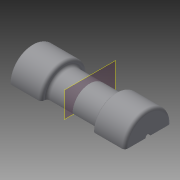
# Autodesk Inventor part: resistor
Saved by Autodesk Inventor 2015 (Build 190159000, 159)
## iProperties
Created: 2014-08-01
Part Number: resistor
Material: Generic
Document SubType Name: Modeling
Designer: dan
Density: 1 g/cm^3
Appearance: Default
Author: dan
Autodesk Inventor part; units mm, degrees
ref_plane "XZ Plane" through (0, 0, 0) normal (0, 1, 0) x (-1, 0, 0)
ref_plane "XY Plane" through (0, 0, 0) normal (0, 0, 1) x (1, 0, 0)
sketch "Sketch1" plane through (0, 0, 0) normal (0, 1, 0) x (-1, 0, 0)
  line L0 (0, 0) -> (0, -12.7)
  line L1 (0, -12.7) -> (-17.78, -12.7)
  line L2 (-17.78, -12.7) -> (-17.78, -9.525)
  line L3 (-17.78, -9.525) -> (-45.72, -9.525)
  line L4 (-45.72, -9.525) -> (-45.72, -12.7)
  line L5 (-45.72, -12.7) -> (-63.5, -12.7)
  line L6 (-63.5, -12.7) -> (-63.5, 0)
  line L7 (-63.5, 0) -> (-60.325, 0)
  line L8 (-60.325, 0) -> (-60.325, -6.35)
  line L9 (-60.325, -6.35) -> (-3.175, -6.35)
  line L10 (-3.175, -6.35) -> (-3.175, 0)
  line L11 (-3.175, 0) -> (0, 0)
  dimension "d0" = 12.7
  dimension "d1" = 3.175
  dimension "d2" = 17.78
  dimension "d3" = 63.5
  dimension "d4" = 3.175
  dimension "d5" = 3.175
  constraints: 24 end point, 10 perpendicular, 3 point on line, 2 collinear, 1 vertical
  measures "d0" distance of L0.start L0.end
  measures "d1" distance of L1.end L2.end
  measures "d2" distance of L0.end L1.end
  measures "d3" distance between parallel lines of L6 L0
  measures "d4" distance between parallel lines of L3 L9
  measures "d5" distance of L10.end L0.start
revolve "Revolution1" add sketch "Sketch1" angle 180 about axis through (63.5, 0, 0) along (1, 0, 0)
fillet "Fillet1" radius 1.5875 6 edges at (63.5, 12.7, 0) (17.78, 9.525, 0) (17.78, 12.7, 0) (0, 12.7, 0) (45.72, 9.525, 0) (45.72, 12.7, 0)
sketch "Sketch2" plane through (0, 0, 0) normal (-1, 0, 0) x (0, 0, 1)
  circle A0 centre (0, 0) radius 1.397
  dimension "d8" = 2.794
  constraints: 1 centre point, 1 coincident
  measures "d8" diameter of A0
extrude "Extrusion1" cut sketch "Sketch2" against normal through all
sketch "Sketch3" plane through (3.175, 0, 6.35) normal (0, -1, 0) x (1, 0, 0)
  line L0 (0, 0) -> (57.15, 0) construction
  line L1 (57.15, -12.7) -> (0, -12.7) construction
  line L2 (0, -4.953) -> (0, -7.747) construction
  line L3 (0, -6.35) -> (10.7724, -6.35) construction
  line L4 (10.7724, -6.35) -> (46.1567, -6.35) construction
  line L5 (46.1567, -6.35) -> (56.929, -6.35) construction
  line L6 (0, -12.7) -> (0, 0) projected
  line L7 (28.575, 0) -> (28.575, -12.7) construction
  line L8 (57.15, -7.747) -> (57.15, -4.953) projected
  line L9 (28.575, -10.7083) -> (28.575, -12.7)
  line L10 (57.15, -7.747) -> (28.575, -7.747) construction
  line L11 (28.575, -10.7083) -> (38.743, -10.7083)
  line L12 (40.775, -8.8314) -> (40.775, -12.7)
  line L13 (40.775, -12.7) -> (28.575, -12.7)
  line L14 (28.575, -12.7) -> (28.575, -10.7083)
  line L15 (38.743, -10.7083) -> (38.743, -12.7)
  line L16 (36.4298, -11.4703) -> (36.4298, -10.7083) construction
  line L17 (29.337, -10.5155) -> (28.575, -10.5155) construction
  line L18 (37.981, -10.5156) -> (38.743, -10.5156) construction
  line L19 (38.743, -10.7083) -> (38.743, -8.8314)
  line L20 (38.743, -8.8314) -> (40.775, -8.8314)
  circle A0 centre (54.9756, -10.5155) radius 1.55
  arc A1 (57.15, -7.747) -> (52.197, -12.7) centre (57.15, -12.7) ccw
  line L21 (57.15, -12.7) -> (53.6477, -9.1977) construction
  line L22 (57.15, -7.747) -> (57.15, -12.7)
  line L23 (57.15, -12.7) -> (52.197, -12.7)
  point P0 (-3.175, -6.35)
  dimension "d27" = 2.032
  dimension "d28" = 3.1
  constraints: 38 end point, 6 perpendicular, 6 point on line, 4 midpoint, 3 equal length, 3 horizontal, 3 point on circle, 2 centre point, 2 parallel, 2 vertical, 1 coincident, 1 collinear, 1 symmetric about line
  measures "d27" distance between parallel lines of L12 L15
  measures "d28" diameter of A0
extrude "Extrusion3" add sketch "Sketch3" against normal up to next
mirror "Mirror1" about plane through (0, 0, 0) normal (0, 0, 1) of "Extrusion3"
ref_plane "Work Plane1" through (31.75, 0, -9.525) normal (1, 0, 0) x (0, 1, 0)
mirror "Mirror2" about plane through (31.75, 0, -9.525) normal (1, 0, 0) of "Extrusion3", "Mirror1"
sketch "Sketch4" plane through (19.3675, 0, -9.525) normal (0, -1, 0) x (1, 0, 0)
  line L0 (22.5505, 3.175) -> (2.2145, 3.175)
  line L1 (2.2145, 3.175) -> (2.2145, 15.8996)
  line L2 (2.2145, 15.8996) -> (22.5505, 15.8996)
  line L3 (22.5505, 15.8996) -> (22.5505, 3.175)
  point P0 (-19.3675, 9.525)
  point P1 (36.0045, 3.175)
  point P2 (40.9575, 3.175)
  point P3 (24.5825, 7.0436)
  constraints: 8 end point, 2 parallel, 1 horizontal, 1 perpendicular
extrude "Extrusion4" cut sketch "Sketch4" against normal blind 1.6002
ref_plane "Work Plane2" through (31.75, 0, -9.525) normal (1, 0, 0) x (0, 1, 0)
body "Solid1"
